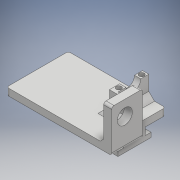
# Autodesk Inventor part: CarroXY - Hotend
Saved by Autodesk Inventor 2017 (Build 210142000, 142)
## iProperties
Created: 2020-08-23
Part Number: CarroXY - Hotend
Material: Generic
Document SubType Name: Modeling
Designer: ale
Density: 1 g/cm^3
Appearance: Default
Author: ale
Autodesk Inventor part; units mm, degrees
ref_plane "YZ Plane" through (0, 0, 0) normal (1, 0, 0) x (0, 1, 0)
ref_plane "XZ Plane" through (0, 0, 0) normal (0, 1, 0) x (-1, 0, 0)
ref_plane "XY Plane" through (0, 0, 0) normal (0, 0, 1) x (1, 0, 0)
sketch "Sketch2" plane through (0, 0, 0) normal (1, 0, 0) x (0, 1, 0)
  line L0 (-19.9252, 0) -> (19.9252, 0)
  line L1 (0, -28.9507) -> (0, 28.9507)
  line L2 (14.5, -7.25) -> (-14.5, -7.25)
  line L3 (-14.5, -7.25) -> (-14.5, -3.25)
  line L4 (-9.5, -3.25) -> (-9.5, 3.25)
  line L5 (-27, 3.25) -> (-27, 9.25)
  line L6 (-27, 9.25) -> (27, 9.25)
  line L7 (14.5, -7.25) -> (14.5, -3.25)
  line L8 (9.5, -3.25) -> (9.5, 3.25)
  line L9 (27, 3.25) -> (27, 9.25)
  line L10 (-14.5, -3.25) -> (-9.5, -3.25)
  line L11 (9.5, -3.25) -> (14.5, -3.25)
  line L12 (27, 3.25) -> (9.5, 3.25)
  line L13 (-9.5, 3.25) -> (-27, 3.25)
  point P0 (0, 0)
  point P1 (0, 0)
  point P2 (9.5, 0)
  dimension "d4" = 14.5
  dimension "d8" = 27
  dimension "d9" = 9.5
  dimension "d10" = 4
  dimension "d11" = 6.5
  dimension "d12" = 6
  constraints: 28 end point, 10 perpendicular, 6 symmetric about line, 3 midpoint, 2 horizontal, 1 coincident, 1 point on line, 1 vertical
  measures "d4" distance between parallel lines of L3 L1
  measures "d8" distance between parallel lines of L5 L1
  measures "d9" distance between parallel lines of L4 L1
  measures "d10" distance between parallel lines of L10 L2
  measures "d11" distance between parallel lines of L13 L10
  measures "d12" distance between parallel lines of L6 L13
extrude "Extrusion2" add sketch "Sketch2" along normal blind 85
sketch "Sketch3" plane through (0, -27, 9.25) normal (0, 0, 1) x (1, 0, 0)
  line L0 (0, 0) -> (85, 0) projected
  line L1 (0, 54) -> (85, 54) projected
  line L2 (65, 27) -> (65, 54)
  line L3 (65, 54) -> (70.5, 54)
  line L4 (70.5, 54) -> (70.5, 27)
  line L5 (85, 54) -> (85, 0) projected
  line L6 (65, 27) -> (70.5, 27)
  point P0 (0, 27)
  dimension "d15" = 20
  dimension "d16" = 5.5
  dimension "d43" = 27
  dimension "d44" = 27
  constraints: 8 end point, 1 point on line
  measures "d15" distance between parallel lines of L5 L2
  measures "d16" distance between parallel lines of L2 L4
  measures "d43" distance from line of L1 L2.start
  measures "d44" distance from line of L1 L4.end
extrude "Extrusion3" add sketch "Sketch3" along normal blind 18
sketch "Sketch7" plane through (0, -27, 3.25) normal (0, 0, -1) x (-1, 0, 0)
  line L0 (-15, 0) -> (55, 0)
  line L1 (-85, 0) -> (-92, 0)
  line L2 (-92, 0) -> (-92, 27)
  line L3 (-92, 27) -> (-85, 27)
  line L4 (-85, 27) -> (-85, 0)
  line L5 (55, 54) -> (55, 0)
  line L6 (-85, 0) -> (-85, 17.5) projected
  point P0 (0, 27)
  dimension "d45" = 7
  dimension "d50" = 0
  constraints: 12 end point, 2 parallel, 1 horizontal, 1 perpendicular, 1 point on line
  measures "d45" distance of L2.end L3.end
  measures "d50" distance between parallel lines of L6 L4
extrude "Extrusion6" add sketch "Sketch7" against normal blind 37
sketch "Sketch9" plane through (65, 0, 9.25) normal (-1, 0, 0) x (0, 0, 1)
  line L0 (18, 27) -> (18, 0) projected
  line L1 (0, -27) -> (31, -27) projected
  point P0 (-9.25, 0)
  point P1 (18, 13.5)
  constraints: 1 midpoint
hole "Hole2" at (65, 13.5, 27.25) direction (1, 0, 0) diameter 13 end through all
sketch "Sketch10" plane through (0, -27, 27.25) normal (0, 0, 1) x (1, 0, 0)
  line L0 (70.5, 54) -> (65, 54) projected
  line L1 (65, 54) -> (65, 47) projected
  line L2 (55.5, 40.5) -> (50, 40.5)
  line L3 (65, 34) -> (65, 47)
  line L4 (85, 54) -> (85, 27) projected
  line L5 (70.5, 54) -> (85, 54) projected
  point P0 (0, 27)
  point P1 (67.75, 50.5)
  point P2 (67.75, 30.5)
  dimension "d99" = 20
  dimension "d100" = 13.5
  dimension "d101" = 2.75
  dimension "d102" = 3.5
  dimension "d103" = 2.75
  dimension "d104" = 23.5
  constraints: 4 end point
  measures "d99" distance between parallel lines of L4 L3
  measures "d100" distance between parallel lines of L2 L5
  measures "d101" distance from line of L1 point (67.75, 50.5)
  measures "d102" distance from line of L0 point (67.75, 50.5)
  measures "d103" distance from line of point (67.75, 30.5) L1
  measures "d104" distance from line of L0 point (67.75, 30.5)
hole "Hole3" at (67.75, 23.5, 27.25) at (67.75, 3.5, 27.25) direction (0, 0, -1) diameter 4.5 end through all
sketch "Sketch11" plane through (0, -14.5, -7.25) normal (0, 0, -1) x (-1, 0, 0)
  circle A0 centre (-67.75, 18) radius 2.25 projected
  line L0 (-71.25, 18) -> (-69.5, 21.0311)
  line L1 (-69.5, 21.0311) -> (-66, 21.0311)
  line L2 (-66, 21.0311) -> (-64.25, 18)
  line L3 (-64.25, 18) -> (-66, 14.9689)
  line L4 (-66, 14.9689) -> (-69.5, 14.9689)
  line L5 (-69.5, 14.9689) -> (-71.25, 18)
  circle A1 centre (-67.75, 38) radius 2.25 projected
  line L6 (-56.25, 38) -> (-54.5, 41.0311)
  line L7 (-54.5, 41.0311) -> (-51, 41.0311)
  line L8 (-51, 41.0311) -> (-49.25, 38)
  line L9 (-49.25, 38) -> (-51, 34.9689)
  line L10 (-51, 34.9689) -> (-54.5, 34.9689)
  line L11 (-54.5, 34.9689) -> (-56.25, 38)
  point P0 (0, 14.5)
  point P1 (-52.75, 38)
  dimension "d71" = 7
  dimension "d74" = 7
  constraints: 24 end point, 2 coincident, 26 other
  measures "d71" distance of L0.start L2.end
  measures "d74" distance of L6.start L9.start
extrude "Extrusion7" cut sketch "Sketch11" against normal blind 14.5 contours L0 L1 L2 L3 L4 L5 | L6 L7 L8 L9 L10 L11
fillet "Fillet1" radius 2 6 edges at (88.5, 0, 40.25) (88.5, -27, 40.25) (85, 27, 6.25) (0, 27, 6.25) (0, -27, 6.25) (92, -13.5, 3.25)
sketch "Sketch13" plane through (65, 0, 9.25) normal (0, -1, 0) x (1, 0, 0)
  line L0 (27, -4) -> (27, 29) projected
  line L1 (0, 18) -> (27, 18)
  line L2 (27, 18) -> (27, 0)
  line L3 (27, 0) -> (0, 0)
  line L4 (0, 0) -> (0, 18)
  point P0 (-65, -9.25)
  point P1 (20, 0)
  dimension "d95" = 0
  constraints: 8 end point, 2 parallel, 1 horizontal, 1 perpendicular, 1 point on line
  measures "d95" distance from line of point (20, 0) L3
extrude "Extrusion9" add sketch "Sketch13" along normal blind 2
chamfer "Chamfer3" distance 5 angle 45 6 edges at (65, 12.5, 9.25) (70.5, 13.5, 9.25) (85, -4.75, 3.25) (85, 0, 6.25) (77.75, 0, 9.25) (75, -2, 9.25)
sketch "Sketch14" plane through (85, -25, 40.25) normal (-1, 0, 0) x (0, 0, 1)
  circle A0 centre (-13, 9.5) radius 9.5
  line L0 (-31, -2) -> (-2, -2) projected
  line L1 (0, 23) -> (0, 0) projected
  point P0 (-40.25, 25)
  point P1 (-26, -2)
  dimension "d85" = 19
  dimension "d86" = 11.5
  dimension "d94" = 13
  constraints: 1 centre point
  measures "d85" diameter of A0
  measures "d86" distance from line of L0 A0.centre
  measures "d94" distance from line of L1 A0.centre
hole "Hole4" at (85, -15.5, 27.25) direction (1, 0, 0) diameter 13.2 end through all
chamfer "Chamfer4" distance 3 angle 45 1 edges at (85, -17, 9.25)
body "Solid2"
